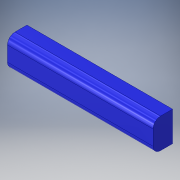
# Autodesk Inventor part: Side Bumper
Saved by Autodesk Inventor 2017 (Build 210142000, 142)
## iProperties
Created: 2017-01-13
Part Number: Side Bumper
Material: Generic
Document SubType Name: Modeling
Designer: Ben
Density: 1 g/cm^3
Appearance: Blue - Wall Paint - Glossy
Author: Ben
Autodesk Inventor part; units mm, degrees
ref_plane "YZ Plane" through (0, 0, 0) normal (1, 0, 0) x (0, 1, 0)
ref_plane "XZ Plane" through (0, 0, 0) normal (0, 1, 0) x (-1, 0, 0)
ref_plane "XY Plane" through (0, 0, 0) normal (0, 0, 1) x (1, 0, 0)
sketch "Sketch1" plane through (0, 0, 0) normal (1, 0, 0) x (0, 1, 0)
  line L0 (0, 0) -> (127, 0)
  line L1 (127, 0) -> (127, 50.8)
  line L2 (0, 0) -> (0, 50.8)
  arc A0 (95.25, 82.55) -> (127, 50.8) centre (95.25, 50.8) ccw construction
  arc A1 (31.75, 82.55) -> (0, 50.8) centre (31.75, 50.8) ccw
  line L3 (95.25, 82.55) -> (31.75, 82.55)
  arc A2 (127, 50.8) -> (95.25, 82.55) centre (95.25, 50.8) ccw
  line L4 (127, 19.05) -> (0, 19.05) construction
  dimension "d0" = 127
  dimension "d1" = 63.5
  dimension "d2" = 19.05
  constraints: 10 end point, 6 point on circle, 5 tangent, 3 centre point, 2 horizontal, 2 point on line, 2 vertical, 1 parallel, 1 perpendicular
  measures "d0" distance of L0.start L0.end
  measures "d1" diameter of A0
  measures "d2" distance between parallel lines of L0 L4
extrude "Extrusion1" add sketch "Sketch1" along normal blind 617.474
body "Solid1"
